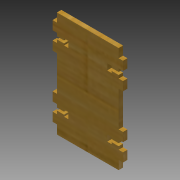
# Autodesk Inventor part: frontal
Saved by Autodesk Inventor 2014 (Build 180170000, 170)
## iProperties
Created: 2015-01-27
Part Number: frontal
Material: Generic
Document SubType Name: Modeling
Designer: Gabriel
Density: 1 g/cm^3
Appearance: Default
Author: Gabriel
Autodesk Inventor part; units mm, degrees
sketch "Sketch1" plane through (0, 0, 0) normal (0, 1, 0) x (-1, 0, 0)
  line L0 (0, -120) -> (70, -120)
  line L1 (70, 0) -> (0, 0)
  line L2 (0, 0) -> (0, -5)
  line L3 (0, -120) -> (0, -115)
  line L4 (0, -5) -> (0, -3.5)
  line L5 (0, -120) -> (0, -115)
  line L6 (70, 45) -> (70, 46.5)
  line L7 (70, -73.5) -> (70, -26.5)
  line L8 (70, -60) -> (70, -58.5)
  line L9 (70, -73.5) -> (70, -88.5)
  line L10 (0, -115) -> (0, -120)
  line L11 (70, -73.5) -> (70, -76.5)
  line L12 (0, -33.5) -> (0, -36.5)
  line L13 (0, -80) -> (0, -36.5)
  line L14 (0, -55) -> (0, -26.5)
  line L15 (0, -26.5) -> (8, -26.5)
  line L16 (8, -26.5) -> (8, -28.5)
  line L17 (8, -28.5) -> (13, -28.5)
  line L18 (13, -28.5) -> (13, -21.5)
  line L19 (13, -21.5) -> (8, -21.5)
  line L20 (8, -21.5) -> (8, -23.5)
  line L21 (8, -23.5) -> (0, -23.5)
  line L22 (13, -25) -> (57, -25)
  line L23 (70, -25) -> (70, -23.5)
  line L24 (70, -23.5) -> (62, -23.5)
  line L25 (62, -23.5) -> (62, -21.5)
  line L26 (62, -21.5) -> (57, -21.5)
  line L27 (57, -21.5) -> (57, -28.5)
  line L28 (57, -28.5) -> (62, -28.5)
  line L29 (62, -28.5) -> (62, -26.5)
  line L30 (62, -26.5) -> (70, -26.5)
  line L31 (0, 0) -> (0, -23.5)
  line L32 (0, -26.5) -> (0, -55)
  line L33 (0, -5) -> (0, -23.5)
  line L34 (0, -26.5) -> (0, -33.5)
  line L35 (0, -5) -> (0, -23.5)
  line L36 (0, -26.5) -> (0, -33.5)
  line L37 (0, 0) -> (0, -23.5)
  line L38 (0, -26.5) -> (0, -33.5)
  line L39 (70, 0) -> (70, -23.5)
  line L40 (70, -26.5) -> (70, -88.5)
  line L41 (0, -83.5) -> (0, -80)
  line L42 (0, -80) -> (0, -83.5)
  line L43 (70, -88.5) -> (70, -76.5)
  line L44 (13, -25) -> (0, -25)
  line L45 (0, -83.5) -> (0, -88.5)
  line L46 (0, -91.5) -> (0, -88.5)
  line L47 (70, -91.5) -> (70, -88.5)
  line L48 (0, -26.5) -> (0, -60)
  line L49 (0, -60) -> (70, -60)
  line L50 (0, -93.5) -> (8, -93.5)
  line L51 (8, -93.5) -> (8, -91.5)
  line L52 (8, -91.5) -> (13, -91.5)
  line L53 (13, -91.5) -> (13, -98.5)
  line L54 (13, -98.5) -> (8, -98.5)
  line L55 (8, -98.5) -> (8, -96.5)
  line L56 (8, -96.5) -> (0, -96.5)
  line L57 (13, -95) -> (57, -95)
  line L58 (70, -96.5) -> (62, -96.5)
  line L59 (62, -96.5) -> (62, -98.5)
  line L60 (62, -98.5) -> (57, -98.5)
  line L61 (57, -98.5) -> (57, -91.5)
  line L62 (57, -91.5) -> (62, -91.5)
  line L63 (62, -91.5) -> (62, -93.5)
  line L64 (62, -93.5) -> (70, -93.5)
  line L65 (0, -93.5) -> (0, -86.5)
  line L66 (0, -93.5) -> (0, -86.5)
  line L67 (0, -93.5) -> (0, -86.5)
  line L68 (0, -91.5) -> (0, -93.5)
  line L69 (0, -96.5) -> (0, -110)
  line L70 (0, -120) -> (0, -96.5)
  line L71 (0, -93.5) -> (0, -91.5)
  line L72 (70, -120) -> (70, -96.5)
  line L73 (70, -93.5) -> (70, -91.5)
  dimension "d70" = 120
  dimension "d115" = 5
  dimension "d116" = 7
  dimension "d117" = 5
  dimension "d119" = 8
  dimension "d120" = 2
  dimension "d121" = 5
  dimension "d123" = 25
  dimension "d124" = 1.5
  dimension "d125" = 1.5
  dimension "d126" = 1.5
  dimension "d127" = 1.5
  dimension "d128" = 35
  dimension "d130" = 70
  dimension "d131" = 8
  dimension "d132" = 2
  constraints: 148 end point, 21 perpendicular, 19 symmetric about line, 10 parallel, 9 collinear, 8 point on line, 4 midpoint, 2 vertical
  measures "d70" distance between parallel lines of L0 L1
  measures "d115" distance of L16.end L17.end
  measures "d116" distance of L17.end L18.end
  measures "d117" distance of L18.end L19.end
  measures "d119" distance of L23.end L24.end
  measures "d120" distance of L24.end L25.end
  measures "d121" distance of L25.end L26.end
  measures "d123" distance between parallel lines of L1 L44
  measures "d124" distance between parallel lines of L44 L21
  measures "d125" distance between parallel lines of L15 L44
  measures "d126" distance between parallel lines of L22 L24
  measures "d127" distance between parallel lines of L30 L22
  measures "d128" distance of L44.end L48.end
  measures "d130" distance between parallel lines of L72 L70
  measures "d131" distance of L14.end L15.end
  measures "d132" distance of L15.end L16.end
ref_plane "Work Plane2" through (0, 0, 0) normal (0, -1, 0) x (1, 0, 0)
sketch "Sketch2" plane through (0, 0, 0) normal (0, -1, 0) x (1, 0, 0)
  point P0 (0, 0)
ref_plane "Work Plane3" through (0, 0, 0) normal (1, 0, 0) x (0, 0, -1)
sketch "Sketch3" plane through (0, 0, 0) normal (1, 0, 0) x (0, 0, -1)
  line L0 (0, 0) -> (10, 0)
  line L1 (10, 0) -> (10, 5)
  line L2 (10, 5) -> (20, 5)
  line L3 (20, 5) -> (20, 0)
  line L4 (20, 0) -> (10, 0)
  line L5 (20, 0) -> (30, 0)
  line L6 (30, 0) -> (30, 5)
  line L7 (30, 5) -> (40, 5)
  line L8 (40, 5) -> (40, 0)
  line L9 (40, 0) -> (30, 0)
  line L10 (40, 0) -> (80, 0)
  line L11 (80, 0) -> (80, 5)
  line L12 (80, 5) -> (90, 5)
  line L13 (90, 5) -> (90, 0)
  line L14 (90, 0) -> (100, 0)
  line L15 (100, 0) -> (100, 5)
  line L16 (100, 5) -> (110, 5)
  line L17 (110, 5) -> (110, 0)
  line L18 (110, 0) -> (100, 0)
  line L19 (90, 0) -> (80, 0)
  dimension "d46" = 10
  dimension "d47" = 5
  dimension "d48" = 10
  dimension "d49" = 10
  dimension "d50" = 10
  dimension "d75" = 5
  dimension "d76" = 10
  dimension "d77" = 10
  dimension "d78" = 5
  dimension "d79" = 10
  dimension "d129" = 40
  constraints: 40 end point, 8 parallel, 6 collinear, 5 perpendicular, 1 horizontal
  measures "d46" distance of L0.start L0.end
  measures "d47" distance of L0.end L1.end
  measures "d48" distance of L1.end L2.end
  measures "d49" distance of L3.end L5.end
  measures "d50" distance of L6.end L7.end
  measures "d75" distance of L10.end L11.end
  measures "d76" distance of L11.end L12.end
  measures "d77" distance of L13.end L14.end
  measures "d78" distance of L14.end L15.end
  measures "d79" distance of L15.end L16.end
  measures "d129" distance between parallel lines of L11 L8
ref_plane "Work Plane1" through (-70, 0, 0) normal (-1, 0, 0) x (0, 0, 1)
sketch "Sketch4" plane through (-70, 0, 0) normal (-1, 0, 0) x (0, 0, 1)
  line L0 (0, 0) -> (-10, 0)
  line L1 (-10, 0) -> (-10, 5)
  line L2 (-10, 5) -> (-20, 5)
  line L3 (-20, 5) -> (-20, 0)
  line L4 (-10, 0) -> (-20, 0)
  line L5 (-20, 0) -> (-30, 0)
  line L6 (-30, 0) -> (-30, 5)
  line L7 (-30, 5) -> (-40, 5)
  line L8 (-40, 5) -> (-40, 0)
  line L9 (-40, 0) -> (-30, 0)
  line L10 (-40, 5) -> (-40, 0)
  line L11 (-40, 0) -> (-80, 0)
  line L12 (-80, 0) -> (-80, 5)
  line L13 (-80, 5) -> (-90, 5)
  line L14 (-90, 5) -> (-90, 0)
  line L15 (-90, 0) -> (-80, 0)
  line L16 (-90, 0) -> (-100, 0)
  line L17 (-100, 0) -> (-100, 5)
  line L18 (-100, 5) -> (-110, 5)
  line L19 (-110, 5) -> (-110, 0)
  line L20 (-100, 0) -> (-110, 0)
  dimension "d58" = 10
  dimension "d59" = 5
  dimension "d60" = 10
  dimension "d61" = 10
  dimension "d62" = 10
  dimension "d80" = 40
  dimension "d81" = 10
  dimension "d82" = 10
  dimension "d83" = 10
  constraints: 42 end point, 14 perpendicular, 4 collinear, 2 parallel, 1 horizontal, 1 point on line
  measures "d58" distance of L0.start L0.end
  measures "d59" distance of L0.end L1.end
  measures "d60" distance of L1.end L2.end
  measures "d61" distance of L3.end L5.end
  measures "d62" distance of L6.end L7.end
  measures "d80" distance of L8.end L11.end
  measures "d81" distance of L12.end L13.end
  measures "d82" distance of L14.end L16.end
  measures "d83" distance of L17.end L18.end
extrude "Extrusion12" add sketch "Sketch1" along normal blind 5
extrude "Extrusion13" add sketch "Sketch3" along normal blind 5
extrude "Extrusion14" add sketch "Sketch4" along normal blind 5
body "Solid2"
